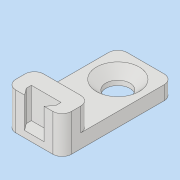
# Autodesk Inventor part: HallEffectSpoolSensorMount
Saved by Autodesk Inventor 2017.3 (Build 213256000, 256)
## iProperties
Created: 2018-04-12
Part Number: HallEffectSpoolSensorMount
Material: ABS Plastic
Document SubType Name: Modeling
Designer: Derek Wider
Density: 1.06 g/cm^3
Appearance: Smooth - White
Author: Derek Wider
Autodesk Inventor part; units mm, degrees
ref_plane "YZ Plane" through (0, 0, 0) normal (1, 0, 0) x (0, 1, 0)
ref_plane "XZ Plane" through (0, 0, 0) normal (0, 1, 0) x (-1, 0, 0)
ref_plane "XY Plane" through (0, 0, 0) normal (0, 0, 1) x (1, 0, 0)
sketch "Sketch1" plane through (0, 0, 0) normal (0, 1, 0) x (-1, 0, 0)
  line L0 (0, 0) -> (7.62, 0)
  line L1 (7.62, 0) -> (7.62, -15.24)
  line L2 (7.62, -15.24) -> (0, -15.24)
  line L3 (0, -15.24) -> (0, 0)
  dimension "d0" = 7.62
  dimension "d1" = 15.24
  constraints: 8 end point, 2 parallel, 1 horizontal, 1 perpendicular
  measures "d0" distance of L0.start L0.end
  measures "d1" distance of L0.end L1.end
extrude "Extrusion1" add sketch "Sketch1" along normal blind 1.905
sketch "Sketch4" plane through (0, 1.905, 0) normal (0, 1, 0) x (1, 0, 0)
  line L0 (0, 15.24) -> (-7.62, 15.24) projected
  circle A0 centre (-3.81, 11.43) radius 1.651
  point P0 (0, 0)
  point P1 (-3.81, 15.24)
  dimension "d9" = 3.302
  dimension "d10" = 3.81
  constraints: 1 centre point, 1 midpoint, 1 vertical alignment
  measures "d9" diameter of A0
  measures "d10" distance of point (-3.81, 15.24) A0.centre
extrude "Extrusion3" cut sketch "Sketch4" against normal through all
chamfer "Chamfer1" distance 1.27 angle 45 1 edges at (-5.461, 1.905, -11.43)
sketch "Sketch5" plane through (0, 1.905, 0) normal (0, 1, 0) x (1, 0, 0)
  line L0 (-7.62, 0) -> (0, 0) projected
  line L1 (0, 0) -> (0, 15.24) projected
  line L2 (0, 15.24) -> (-7.62, 15.24) projected
  line L3 (-7.62, 15.24) -> (-7.62, 0) projected
  circle A0 centre (-3.81, 11.43) radius 2.921 projected
  line L4 (0, 0) -> (-7.62, 0) projected
  line L5 (-5.1435, 0) -> (-5.842, 0.9271)
  line L6 (-5.842, 0.9271) -> (-5.842, 1.6256)
  line L7 (-5.842, 1.6256) -> (-1.778, 1.6256)
  line L8 (-1.778, 1.6256) -> (-1.778, 0.9271)
  line L9 (-1.778, 0.9271) -> (-2.4765, 0)
  line L10 (-7.62, 0) -> (-7.62, 15.24) projected
  line L11 (-7.62, 3.81) -> (0, 3.81)
  point P0 (-3.81, 1.6256)
  point P1 (-3.81, 3.81)
  dimension "d19" = 2.667
  dimension "d20" = 4.064
  dimension "d21" = 0.9271
  dimension "d23" = 1.6256
  dimension "d24" = 3.81
  constraints: 12 end point, 4 perpendicular, 4 point on line, 2 midpoint, 1 equal length, 1 horizontal alignment, 1 vertical alignment
  measures "d19" distance of L9.end L5.start
  measures "d20" distance of L6.end L7.end
  measures "d21" vertical distance of L9.end L8.end
  measures "d23" distance between parallel lines of L0 L7
  measures "d24" distance between parallel lines of L0 L11
extrude "Extrusion4" add sketch "Sketch5" along normal blind 3.175 contours L3 L11 L1 L0 L9 L8 L7 L6 L5
fillet "Fillet2" radius 1.27 6 edges at (-7.62, 2.54, 0) (0, 2.54, 0) (0, 3.4925, -3.81) (-7.62, 3.4925, -3.81) (-7.62, 0.9525, -15.24) (0, 0.9525, -15.24)
sketch "Sketch6" plane through (0, 1.905, 0) normal (0, 1, 0) x (1, 0, 0)
  line L0 (-2.4765, 0) -> (-1.778, 0.9271) projected
  line L1 (-1.778, 0.9271) -> (-1.778, 1.6256) projected
  line L2 (-1.778, 1.6256) -> (-5.842, 1.6256) projected
  line L3 (-5.842, 1.6256) -> (-5.842, 0.9271) projected
  line L4 (-5.842, 0.9271) -> (-5.1435, 0) projected
  line L5 (-5.1435, 0) -> (-2.4765, 0) projected
  point P0 (0, 0)
extrude "Extrusion5" cut sketch "Sketch6" against normal blind 1.016
body "Solid1"
